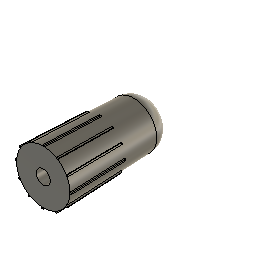
CsabiKertiSzekStift2 (Autodesk Fusion 360 design; units mm, degrees)
part number: 2026-06-04-21-25-07-122
Autodesk Fusion 360 part; units mm, degrees
sketch "Sketch1" plane through (0, 0, 0) normal (0, 0, 1) x (1, 0, 0)
  line L0 (0, 0) -> (4.75, 0)
  line L1 (4.75, 0) -> (4.1138, 16.1183)
  line L2 (1.1161, 19) -> (0, 19)
  line L3 (0, 19) -> (0, 0)
  arc A0 (4.1138, 16.1183) -> (1.1161, 19) centre (1.1161, 16) ccw
  point P0 (4, 19)
  dimension "d5" = 19
  dimension "d6" = 4.75
  dimension "d7" = 4
  dimension "d8" = 3
  constraint horizontal L0
  constraint parallel L0 L2
  constraint perpendicular L0 L3
  constraint coincident P0 L1
  constraint coincident P0 L2
  constraint tangent L1 A0
  constraint tangent L2 A0
  constraint coincident L0.start L3.end
  measures "d5" distance of L0.start L2.end
  measures "d6" distance of L0.start L0.end
  measures "d7" distance of P0 L2.end
  measures "d8" radius of A0
revolve "Revolve1" add sketch "Sketch1" angle 360 about axis through (0, 19, 0) along (0, -1, 0)
sketch "Sketch3" plane through (0, 0, 0) normal (0, -1, 0) x (1, 0, 0)
  circle A0 centre (0, 0) radius 1.25
  circle A1 centre (0, 0) radius 4.75
  dimension "d17" = 2.5
  constraint concentric A0 A1
  measures "d17" diameter of A0
ref_plane "WorkPlane1" through (-4.4319, 8.0592, 0) normal (-0.999222, 0.039443, 0) x (0, 0, 1)
sketch "Sketch4" plane through (-4.7426, 0.1872, 0) normal (-0.999222, 0.039443, 0) x (0, 0, 1)
  line L0 (0, 0) -> (0.25, 0)
  line L1 (0.25, 0) -> (0.25, 10)
  line L2 (0.25, 10) -> (0, 10)
  line L3 (0, 10) -> (0, 0)
  dimension "d19" = 0.25
  dimension "d20" = 10
  constraint horizontal L0
  constraint vertical L1
  constraint horizontal L2
  constraint vertical L3
  constraint coincident L0.start L3.end
  measures "d19" distance of L0.start L0.end
  measures "d20" distance of L0.start L2.end
extrude "Extrude2" add sketch "Sketch4" along normal blind 0.25
fillet "Fillet2" radius 0.25 1 edges at (-4.598, 10.1893, 0.125)
extrude "Extrude3" add 1 faces at (-4.9091, 0.1938, 0.1667) along direction (-0.039443, -0.999222, 0) up to surface end surface through (0, 0, 0) normal (0, -1, 0) offset 0
pattern_circular "C-Pattern2" count 12 over 360 about axis through (0, 31.1447, 0) along (0, -1, 0) of "Extrude2", "Fillet2", "Extrude3"
extrude "Extrude4" cut sketch "Sketch3" against normal blind 15 contours A0
equation "d6 = ( 9.5 / 2 ) * 1 mm"
equation "d7 = ( 8 / 2 ) * 1 mm"
named bodies: "Body"
